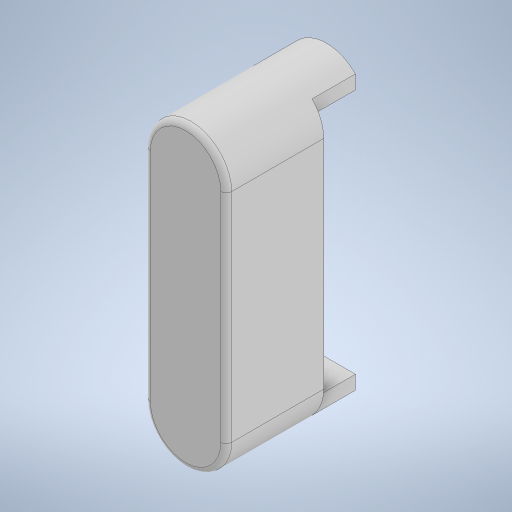
# Autodesk Inventor part: Tapa carcasa Luis
Saved by Autodesk Inventor 2023.4 (Build 274418000, 418)
## iProperties
Created: 2024-01-25
Part Number: Tapa carcasa Luis
Material: Genérico
Document SubType Name: Modeling
Designer: Adrián Álvarez
Density: 1 g/cm^3
Appearance: Valor por defecto
Author: Adrián Álvarez
Autodesk Inventor part; units mm, degrees
ref_plane "YZ Plane" through (0, 0, 0) normal (1, 0, 0) x (0, 1, 0)
ref_plane "XZ Plane" through (0, 0, 0) normal (0, 1, 0) x (-1, 0, 0)
ref_plane "XY Plane" through (0, 0, 0) normal (0, 0, 1) x (1, 0, 0)
sketch "Boceto1" plane through (0, 0, 0) normal (0, 0, 1) x (1, 0, 0)
  line L0 (0, 0) -> (0, 40.1) construction
  line L1 (7.5, 0) -> (7.5, 40.1)
  line L2 (-7.5, 40.1) -> (-7.5, 0)
  arc A0 (-7.5, 0) -> (7.5, 0) centre (0, 0) ccw
  arc A1 (7.5, 40.1) -> (-7.5, 40.1) centre (0, 40.1) ccw
  point P0 (0, 20.05)
  dimension "d0" = 40.1
  dimension "d1" = 15
  constraints: 8 end point, 4 point on circle, 4 tangent, 2 centre point, 1 midpoint, 1 parallel, 1 vertical
  measures "d0" distance of L0.start L0.end
  measures "d1" diameter of A1
extrude "Extrusión1" add sketch "Boceto1" along normal blind 18
sketch "Boceto2" plane through (0, 0, 0) normal (0, 0, -1) x (-1, 0, 0)
  arc A0 (7.5, 40.1) -> (-7.5, 40.1) centre (0, 40.1) ccw projected
  line L0 (0, 40.1) -> (0, 24.6)
  line L1 (0, 24.6) -> (-3.5, 24.6)
  line L2 (-3.5, 24.6) -> (3.5, 24.6)
  line L3 (3.5, 24.6) -> (3.5, 40.1)
  line L4 (3.5, 40.1) -> (-3.5, 40.1)
  line L5 (-3.5, 40.1) -> (-3.5, 24.6)
  point P0 (0, 0)
  dimension "d4" = 15.5
  dimension "d5" = 3.5
  dimension "d6" = 7
  constraints: 12 end point, 4 perpendicular, 1 point on line, 1 vertical
  measures "d4" distance of L0.start L0.end
  measures "d5" distance of L0.end L1.end
  measures "d6" distance of L1.end L2.end
extrude "Extrusión2" cut sketch "Boceto2" against normal blind 17
sketch "Boceto3" plane through (0, 0, 0) normal (0, 0, -1) x (-1, 0, 0)
  line L0 (-3.5, 40.1) -> (3.5, 40.1) projected
  line L1 (0, 40.1) -> (0, 41.1)
  line L2 (7.5, 40.1) -> (7.5, 0) projected
  line L3 (7.5, 20.05) -> (-7.5, 20.05)
  line L4 (-7.5, 0) -> (-7.5, 40.1) projected
  line L5 (0, 0) -> (0, -1)
  line L6 (-5.3571, 42.7751) -> (-5.3571, 44.0501)
  line L7 (-5.3571, -2.6751) -> (-5.3571, -3.9501)
  line L8 (-5.3571, 44.0501) -> (-5.3571, 45.3489)
  arc A0 (7.5, 40.1) -> (-7.5, 40.1) centre (0, 40.1) ccw projected
  arc A1 (5.3571, 45.3489) -> (-5.3571, 45.3489) centre (0, 40.1) ccw
  arc A2 (-5.3571, -5.2489) -> (5.3571, -5.2489) centre (0, 0) ccw
  line L9 (-5.3571, -3.9501) -> (-5.3571, -5.2489)
  line L10 (5.3571, -4.6499) -> (5.3571, -5.2489)
  arc A3 (-7.5, 0) -> (7.5, 0) centre (0, 0) ccw projected
  line L11 (5.3571, 45.3489) -> (5.3571, 42.7751)
  line L12 (-5.3571, 42.7751) -> (5.3571, 42.7751)
  line L13 (5.3571, -4.6499) -> (5.3571, -2.6751)
  line L14 (-5.3571, -2.6751) -> (5.3571, -2.6751)
  point P0 (4.6429, 42.4001)
  dimension "d10" = 1
  constraints: 28 end point, 8 vertical, 7 point on circle, 3 midpoint, 2 centre point, 2 coincident, 2 symmetric about line
  measures "d10" distance of L1.start L1.end
extrude "Extrusión3" add sketch "Boceto3" along normal blind 8 contours L11 L12 L6 L8 A0 | A2 L9 L7 L14 L13 L10
sketch "Boceto4" plane through (0, 0, 0) normal (0, 0, -1) x (-1, 0, 0)
  line L0 (2.5, 24.6) -> (2.5, -1)
  line L1 (2.5, -1) -> (-2.5, -1)
  line L2 (-2.5, -1) -> (-2.5, 24.6)
  line L3 (-2.5, 24.6) -> (2.5, 24.6)
  line L4 (3.5, 24.6) -> (-3.5, 24.6) projected
  point P0 (0, 0)
  constraints: 8 end point, 2 perpendicular, 1 collinear
extrude "Extrusión4" cut sketch "Boceto4" against normal blind 5
fillet "Empalme1" radius 1 4 edges at (0, 47.6, 18) (-7.5, 20.05, 18) (0, -7.5, 18) (7.5, 20.05, 18)
